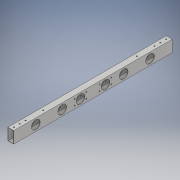
# Autodesk Inventor part: driveline 1x2
Saved by Autodesk Inventor 2018 (Build 220112000, 112)
## iProperties
Created: 2020-03-30
Part Number: driveline 1x2
Material: Generic
Document SubType Name: Modeling
Designer: maste
Density: 1 g/cm^3
Appearance: Default
Author: maste
Autodesk Inventor part; units mm, degrees
ref_plane "YZ Plane" through (0, 0, 0) normal (1, 0, 0) x (0, 1, 0)
ref_plane "XZ Plane" through (0, 0, 0) normal (0, 1, 0) x (-1, 0, 0)
ref_plane "XY Plane" through (0, 0, 0) normal (0, 0, 1) x (1, 0, 0)
sketch "Sketch1" plane through (0, 0, 0) normal (0, 0, 1) x (1, 0, 0)
  line L0 (0, 0) -> (25.4, 0)
  line L1 (25.4, 0) -> (25.4, 50.8)
  line L2 (25.4, 50.8) -> (0, 50.8)
  line L3 (0, 50.8) -> (0, 0)
  line L4 (1.5875, 49.2125) -> (23.8125, 49.2125)
  line L5 (23.8125, 49.2125) -> (23.8125, 1.5875)
  line L6 (23.8125, 1.5875) -> (1.5875, 1.5875)
  line L7 (1.5875, 1.5875) -> (1.5875, 49.2125)
  dimension "d0" = 25.4
  dimension "d1" = 50.8
  dimension "d2" = 1.5875
  constraints: 16 end point, 4 parallel, 2 perpendicular, 1 horizontal, 3 other
  measures "d0" distance of L2.end L1.end
  measures "d1" distance of L1.end L0.end
  measures "d2" distance between parallel lines of L2 L4
extrude "Extrusion1" add sketch "Sketch1" along normal blind 685.8
sketch "Sketch2" plane through (25.4, 0, 0) normal (1, 0, 0) x (0, 0, -1)
  line L0 (0, 49.2125) -> (0, 1.5875) construction
  line L1 (0, 25.4) -> (-95.25, 25.4) construction
  line L2 (0, 25.4) -> (-209.55, 25.4) construction
  line L3 (0, 25.4) -> (-288.925, 25.4) construction
  circle A0 centre (-95.25, 25.4) radius 19.05
  circle A1 centre (-209.55, 25.4) radius 19.05
  circle A2 centre (-288.925, 25.4) radius 19.05
  line L4 (0, 50.8) -> (-685.8, 50.8) construction
  line L5 (-342.9, 50.8) -> (-342.9, -48.6328) construction
  circle A3 centre (-590.55, 25.4) radius 19.05
  circle A4 centre (-476.25, 25.4) radius 19.05
  circle A5 centre (-396.875, 25.4) radius 19.05
  point P0 (0, 0)
  dimension "d5" = 95.25
  dimension "d6" = 209.55
  dimension "d7" = 288.925
  dimension "d8" = 38.1
  dimension "d9" = 38.1
  dimension "d10" = 38.1
  constraints: 8 end point, 6 centre point, 3 coincident, 3 horizontal, 3 symmetric about line, 2 midpoint, 1 vertical, 3 other
  measures "d5" distance of L1.start L1.end
  measures "d6" distance of L1.start L2.end
  measures "d7" distance of L1.start L3.end
  measures "d8" diameter of A0
  measures "d9" diameter of A1
  measures "d10" diameter of A2
extrude "Extrusion2" cut sketch "Sketch2" against normal blind 685.8
sketch "Sketch3" plane through (0, 50.8, 0) normal (0, 1, 0) x (1, 0, 0)
  line L0 (23.8125, 0) -> (1.5875, 0) construction
  line L1 (12.7, 0) -> (12.7, -38.1) construction
  line L2 (12.7, -38.1) -> (12.7, -63.5) construction
  line L3 (12.7, -63.5) -> (12.7, -139.7) construction
  line L4 (25.4, -685.8) -> (0, -685.8) construction
  line L5 (12.7, -685.8) -> (12.7, -647.7) construction
  line L6 (12.7, -647.7) -> (12.7, -622.3) construction
  line L7 (12.7, -622.3) -> (12.7, -546.1) construction
  circle A0 centre (12.7, -647.7) radius 2.5797
  circle A1 centre (12.7, -622.3) radius 2.5797
  circle A2 centre (12.7, -546.1) radius 2.5797
  circle A3 centre (12.7, -139.7) radius 2.5797
  circle A4 centre (12.7, -63.5) radius 2.5797
  circle A5 centre (12.7, -38.1) radius 2.5797
  line L8 (12.7, -685.8) -> (12.7, -673.1) construction
  line L9 (12.7, 0) -> (12.7, -12.7) construction
  circle A6 centre (12.7, -12.7) radius 2.5797
  circle A7 centre (12.7, -673.1) radius 2.5797
  point P0 (0, 0)
  dimension "d13" = 38.1
  dimension "d14" = 25.4
  dimension "d15" = 76.2
  dimension "d16" = 38.1
  dimension "d17" = 25.4
  dimension "d18" = 76.2
  dimension "d19" = 5.1594
  dimension "d24" = 12.7
  dimension "d25" = 12.7
  constraints: 16 end point, 8 centre point, 8 coincident, 6 point on line, 2 midpoint, 2 vertical
  measures "d13" distance of L1.start L1.end
  measures "d14" distance of L1.end L2.end
  measures "d15" distance of L2.end L3.end
  measures "d16" distance of L5.start L5.end
  measures "d17" distance of L5.end L6.end
  measures "d18" distance of L6.end L7.end
  measures "d19" diameter of A0
  measures "d24" distance of L5.start L8.end
  measures "d25" distance of L1.start L9.end
extrude "Extrusion5" cut sketch "Sketch3" against normal blind 215.9
sketch "Sketch4" plane through (25.4, 0, 0) normal (1, 0, 0) x (0, 0, -1)
  line L0 (-685.8, 0) -> (-422.3766, 0) construction
  line L1 (0, 0) -> (-685.8, 0) construction
  line L2 (-422.3766, 0) -> (-422.3766, 12.8524) construction
  line L3 (-422.3766, 12.8524) -> (-422.3766, 38.2524) construction
  line L4 (-422.3766, 38.2524) -> (-371.5766, 38.2524) construction
  line L5 (-371.5766, 38.2524) -> (-371.5766, 12.8524) construction
  line L6 (0, 50.8) -> (-685.8, 50.8) construction
  line L7 (-342.9, 50.8) -> (-342.9, 0) construction
  circle A0 centre (-422.3766, 38.2524) radius 2.5781
  circle A1 centre (-422.3766, 12.8524) radius 2.5781
  circle A2 centre (-371.5766, 12.8524) radius 2.5781
  circle A3 centre (-371.5766, 38.2524) radius 2.5781
  circle A4 centre (-263.4234, 38.2524) radius 2.5781
  circle A5 centre (-263.4234, 12.8524) radius 2.5781
  circle A6 centre (-314.2234, 12.8524) radius 2.5781
  circle A7 centre (-314.2234, 38.2524) radius 2.5781
  dimension "d16" = 38.1
  dimension "d17" = 25.4
  dimension "d18" = 76.2
  dimension "d19" = 5.1594
  dimension "d24" = 12.7
  dimension "d28" = 263.4234
  dimension "d29" = 12.8524
  dimension "d30" = 25.4
  dimension "d31" = 50.8
  dimension "d32" = 25.4
  dimension "d33" = 5.1562
  constraints: 12 end point, 8 centre point, 4 coincident, 4 symmetric about line, 3 perpendicular, 2 midpoint, 2 point on line, 4 other
  measures "d28" distance of L0.start L0.end
  measures "d29" distance of L0.end L2.end
  measures "d30" distance of L2.end L3.end
  measures "d31" distance of L3.end L4.end
  measures "d32" distance of L4.end L5.end
  measures "d33" diameter of A0
extrude "Extrusion6" cut sketch "Sketch4" against normal blind 215.9
body "Solid1"
